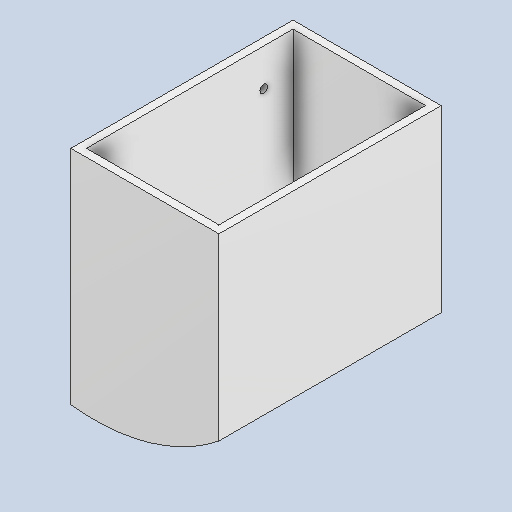
# Autodesk Inventor part: ashish1
Saved by Autodesk Inventor 2022 (Build 260153070, 153G)
## iProperties
Created: 2021-07-03
Part Number: ashish1
Material: PBT Plastic
Document SubType Name: Modeling
Designer: 91852
Density: 1.31 g/cm^3
Appearance: Smooth - White
Author: 91852
Autodesk Inventor part; units mm, degrees
ref_plane "YZ Plane" through (0, 0, 0) normal (1, 0, 0) x (0, 1, 0)
ref_plane "XZ Plane" through (0, 0, 0) normal (0, 1, 0) x (-1, 0, 0)
ref_plane "XY Plane" through (0, 0, 0) normal (0, 0, 1) x (1, 0, 0)
sketch "Sketch1" plane through (0, 0, 0) normal (0, 0, 1) x (1, 0, 0)
  line L0 (0, 9.6698) -> (0, -104.6302)
  line L1 (0, 9.6698) -> (76.2, 9.6698)
  line L2 (76.2, 9.6698) -> (76.2, -82.6078)
  arc A0 (0, -104.6302) -> (76.2, -82.6078) centre (11.8217, -2.6932) ccw
  point P0 (0, 0)
  dimension "d0" = 114.3
  dimension "d1" = 76.2
  constraints: 6 end point, 2 point on circle, 1 centre point, 1 perpendicular, 1 vertical
  measures "d0" distance of L0.start L0.end
  measures "d1" distance of L0.start L1.end
extrude "Extrusion1" add sketch "Sketch1" along normal blind 114.3
sketch "Sketch2" plane through (0, 9.6698, 0) normal (0, 1, 0) x (1, 0, 0)
  line L0 (72.2, -4) -> (4, -4)
  line L1 (4, -4) -> (4, -110.3)
  line L2 (4, -110.3) -> (72.2, -110.3)
  line L3 (72.2, -110.3) -> (72.2, -4)
  line L4 (76.2, -114.3) -> (0, -114.3) projected
  line L5 (76.2, 0) -> (0, 0) projected
  line L6 (76.2, 0) -> (76.2, -114.3) projected
  line L7 (0, 0) -> (0, -114.3) projected
  dimension "d4" = 4
  dimension "d5" = 4
  dimension "d6" = 4
  dimension "d7" = 4
  constraints: 8 end point, 2 parallel, 1 horizontal, 1 perpendicular
  measures "d4" distance between parallel lines of L4 L2
  measures "d5" distance between parallel lines of L5 L0
  measures "d6" distance between parallel lines of L6 L3
  measures "d7" distance between parallel lines of L7 L1
extrude "Extrusion2" cut sketch "Sketch2" against normal blind 90 contours L3 L2 L1 L0
sketch "Sketch3" plane through (0, -104.6302, 0) normal (-1, 0, 0) x (0, 0, 1)
  circle A0 centre (19.05, 95.25) radius 2
  circle A1 centre (95.25, 95.25) radius 2
  circle A2 centre (19.05, 19.05) radius 2
  circle A3 centre (95.25, 19.05) radius 2
  line L0 (0, 114.3) -> (114.3, 114.3) projected
  line L1 (0, 114.3) -> (0, 0) projected
  line L2 (114.3, 114.3) -> (114.3, 0) projected
  line L3 (0, 0) -> (114.3, 0) projected
  point P0 (0, 104.6302)
  dimension "d10" = 4
  dimension "d11" = 4
  dimension "d12" = 4
  dimension "d13" = 4
  dimension "d14" = 19.05
  dimension "d15" = 19.05
  dimension "d16" = 19.05
  dimension "d17" = 19.05
  dimension "d18" = 19.05
  dimension "d19" = 19.05
  dimension "d20" = 19.05
  dimension "d21" = 19.05
  constraints: 4 centre point
  measures "d10" diameter of A0
  measures "d11" diameter of A1
  measures "d12" diameter of A2
  measures "d13" diameter of A3
  measures "d14" distance from line of L0 A0.centre
  measures "d15" distance from line of L1 A0.centre
  measures "d16" distance from line of L0 A1.centre
  measures "d17" distance from line of L2 A1.centre
  measures "d18" distance from line of L1 A2.centre
  measures "d19" distance from line of L3 A2.centre
  measures "d20" distance from line of L2 A3.centre
  measures "d21" distance from line of L3 A3.centre
extrude "Extrusion3" cut sketch "Sketch3" against normal blind 4 contours A0 | A1 | A2 | A3
equation "\"d22\" = d12"
body "Solid1"
